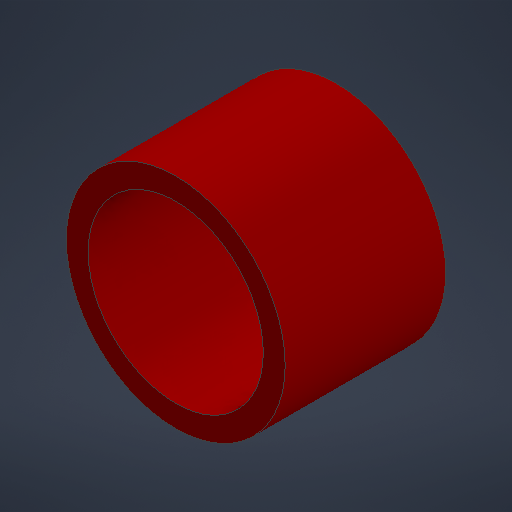
# Autodesk Inventor part: bublegum
Saved by Autodesk Inventor 2025.3 (Build 293356000, 356)
## iProperties
Created: 2025-10-30
Part Number: bublegum
Material: Všeobecné
Document SubType Name: Modeling
Designer: Mr.Happy
Density: 1 g/cm^3
Appearance: Výchozí
Author: Mr.Happy
Autodesk Inventor part; units mm, degrees
ref_plane "YZ Plane" through (0, 0, 0) normal (1, 0, 0) x (0, 1, 0)
ref_plane "XZ Plane" through (0, 0, 0) normal (0, 1, 0) x (-1, 0, 0)
ref_plane "XY Plane" through (0, 0, 0) normal (0, 0, 1) x (1, 0, 0)
sketch "Náčrt1" plane through (0, 0, 0) normal (0, 0, 1) x (1, 0, 0)
  line L0 (0, 22) -> (0, 0)
  line L1 (12, 22) -> (15, 22)
  line L2 (15, 22) -> (15, 0)
  line L3 (15, 0) -> (12, 0)
  line L4 (12, 0) -> (12, 22)
  dimension "d0" = 22
  dimension "d1" = 3
  dimension "d2" = 24
  constraints: 10 end point, 2 horizontal alignment, 2 parallel, 1 horizontal, 1 perpendicular, 1 vertical
  measures "d0" distance of L0.start L0.end
  measures "d1" distance of L2.end L3.end
  measures "d2" diameter of L4 L0
revolve "Rotace1" add sketch "Náčrt1" angle 360 about axis through (0, 22, 0) along (0, -1, 0)
